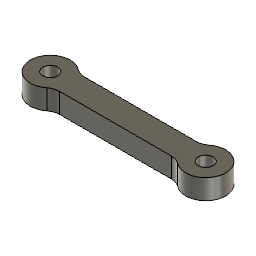
Link (Autodesk Fusion 360 design; units mm, degrees)
part number: 2026-08-19-23-00-53-516
Autodesk Fusion 360 part; units mm, degrees
sketch "Sketch1" plane through (0, 0, 0) normal (0, 0, 1) x (1, 0, 0)
  line L0 (-15.5, 0) -> (15.5, 0) construction
  circle A0 centre (-15.5, 0) radius 1.5
  circle A1 centre (-15.5, 0) radius 4
  circle A2 centre (15.5, 0) radius 1.5
  circle A3 centre (15.5, 0) radius 4
  line L1 (12.3775, -2.5) -> (-12.3775, -2.5)
  line L2 (-12.3775, -2.5) -> (-12.3775, 2.5)
  line L3 (-12.3775, 2.5) -> (12.3775, 2.5)
  line L4 (12.3775, 2.5) -> (12.3775, -2.5)
  line L5 (12.3775, -2.5) -> (-12.3775, 2.5) construction
  line L6 (-12.3775, -2.5) -> (12.3775, 2.5) construction
  line L7 (12.3775, -2.5) -> (13.2, -2.5) construction
  line L8 (12.3775, 2.5) -> (12.9, 2.5) construction
  point P0 (12.3775, -2.5)
  point P1 (12.3775, 2.5)
  dimension "d1" = 31
  dimension "d2" = 3
  dimension "d3" = 8
  dimension "d4" = 3
  dimension "d5" = 8
  dimension "d6" = 5
  constraint midpoint L0 origin
  constraint horizontal L0
  constraint coincident L0.start A0.centre
  constraint concentric A0 A1
  constraint coincident L0.end A2.centre
  constraint concentric A2 A3
  constraint horizontal L1
  constraint perpendicular L1 L2
  constraint parallel L1 L3
  constraint parallel L2 L4
  constraint coincident L5 origin
  constraint coincident L6 origin
  constraint perpendicular L4 L7
  constraint perpendicular L4 L8
  constraint coincident L7 P0
  constraint coincident A3 P0
  constraint coincident A3 P1
  constraint coincident L8 P1
  constraint coincident P0 L1.start
  measures "d1" distance of L0.start L0.end
  measures "d2" diameter of A0
  measures "d3" diameter of A1
  measures "d4" diameter of A2
  measures "d5" diameter of A3
  measures "d6" distance of L1 L3
extrude "Extrude1" add sketch "Sketch1" along normal blind 4
fillet "Fillet1" radius 3 4 edges at (-12.3775, -2.5, 2) (12.3775, -2.5, 2) (12.3775, 2.5, 2) (-12.3775, 2.5, 2)
